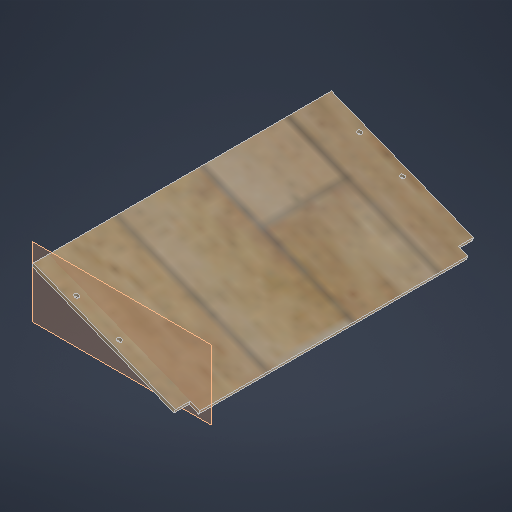
# Autodesk Inventor part: Slope_Riner
Saved by Autodesk Inventor 2026.3 (Build 303398000, 398)
## iProperties
Created: 2026-09-07
Part Number: Slope_Riner
Material: 木材 (カエデ材)
Document SubType Name: Modeling
Designer: takuya
Density: 0.67 g/cm^3
Appearance: ナチュラル カエデ材 - 光沢 濃い着色
Author: takuya
Autodesk Inventor part; units mm, degrees
ref_plane "YZ Plane" through (0, 0, 0) normal (1, 0, 0) x (0, 1, 0)
ref_plane "XZ Plane" through (0, 0, 0) normal (0, 1, 0) x (-1, 0, 0)
ref_plane "XY Plane" through (0, 0, 0) normal (0, 0, 1) x (1, 0, 0)
sketch "スケッチ1" plane through (0, 0, 0) normal (0, 0, 1) x (1, 0, 0)
  line L0 (-53.8577, -21) -> (53.8577, -21) projected
  line L1 (53.8577, -21) -> (53.8577, -19.5) projected
  line L2 (53.8577, -19.5) -> (45.423, -16.1743) projected
  line L3 (45.423, -16.1743) -> (44.506, -18.5) projected
  line L4 (44.506, -18.5) -> (-49.7747, 18.6743) projected
  line L5 (-49.7747, 18.6743) -> (-48.8577, 21) projected
  line L6 (-48.8577, 21) -> (-53.8577, 21) projected
  line L7 (-53.8577, 21) -> (-53.8577, -21) projected
  line L8 (-42.0411, 10.2503) -> (14.7433, -12.1394) projected
  arc A0 (14.0097, -16) -> (14.7433, -12.1394) centre (14.0097, -14) ccw projected
  line L9 (14.0097, -16) -> (-42.7747, -16) projected
  arc A1 (-44.7747, -14) -> (-42.7747, -16) centre (-42.7747, -14) ccw projected
  line L10 (-44.7747, -14) -> (-44.7747, 8.3897) projected
  arc A2 (-42.0411, 10.2503) -> (-44.7747, 8.3897) centre (-42.7747, 8.3897) ccw projected
  line L11 (-48.8577, 21) -> (45.423, -16.1743)
  point P0 (0, 0)
  constraints: 2 end point, 1 perpendicular
extrude "押し出し1" add sketch "スケッチ1" against normal blind 198 contours L11 L3 L4 L5
ref_plane "作業平面1" through (0, 0, -10) normal (0, 0, 1) x (1, 0, 0)
sketch "スケッチ2" plane through (0, 0, 0) normal (0, 0, 1) x (1, 0, 0)
  line L0 (-53.8577, -21) -> (53.8577, -21) projected
  line L1 (53.8577, -21) -> (53.8577, -19.5) projected
  line L2 (53.8577, -19.5) -> (45.423, -16.1743) projected
  line L3 (45.423, -16.1743) -> (44.506, -18.5) projected
  line L4 (44.506, -18.5) -> (-49.7747, 18.6743) projected
  line L5 (-49.7747, 18.6743) -> (-48.8577, 21) projected
  line L6 (-48.8577, 21) -> (-53.8577, 21) projected
  line L7 (-53.8577, 21) -> (-53.8577, -21) projected
  line L8 (-42.0411, 10.2503) -> (14.7433, -12.1394) projected
  arc A0 (14.0097, -16) -> (14.7433, -12.1394) centre (14.0097, -14) ccw projected
  line L9 (14.0097, -16) -> (-42.7747, -16) projected
  arc A1 (-44.7747, -14) -> (-42.7747, -16) centre (-42.7747, -14) ccw projected
  line L10 (-44.7747, -14) -> (-44.7747, 8.3897) projected
  arc A2 (-42.0411, 10.2503) -> (-44.7747, 8.3897) centre (-42.7747, 8.3897) ccw projected
  line L11 (45.423, -16.1743) -> (44.506, -18.5)
  line L12 (44.506, -18.5) -> (50.8464, -21)
  line L13 (50.8464, -21) -> (51.7634, -18.6743)
  line L14 (51.7634, -18.6743) -> (45.423, -16.1743)
  point P0 (0, 0)
  constraints: 8 end point, 2 parallel, 2 perpendicular
extrude "押し出し2" add sketch "スケッチ2" against normal blind 178 from surface at -10 contours L12 L3 L2 L13
sketch "スケッチ3" plane through (-48.8577, 21, 0) normal (0.3668, 0.9303, 0) x (0.9303, -0.3668, 0)
  circle A0 centre (56.0638, 5) radius 1.5 projected
  circle A1 centre (25.5443, 5) radius 1.5 projected
  circle A2 centre (25.5443, 193) radius 1.5 projected
  circle A3 centre (56.0638, 193) radius 1.5 projected
  point P0 (53.1551, 0)
extrude "押し出し3" cut sketch "スケッチ3" against normal blind 2.5
